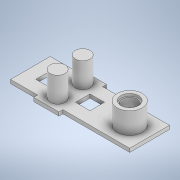
# Autodesk Inventor part: VexLegoWidget2
Saved by Autodesk Inventor 2020 (Build 240168000, 168)
## iProperties
Created: 2020-02-28
Part Number: VexLegoWidget2
Material: Generic
Document SubType Name: Modeling
Designer: Luke
Density: 1 g/cm^3
Appearance: Default
Author: Luke
Autodesk Inventor part; units mm, degrees
ref_plane "YZ Plane" through (0, 0, 0) normal (1, 0, 0) x (0, 1, 0)
ref_plane "XZ Plane" through (0, 0, 0) normal (0, 1, 0) x (-1, 0, 0)
ref_plane "XY Plane" through (0, 0, 0) normal (0, 0, 1) x (1, 0, 0)
sketch "Sketch4" plane through (0, 0, 0) normal (0, 1, 0) x (-1, 0, 0)
  line L0 (-19.05, 6.35) -> (2.3114, 6.35)
  line L1 (19.05, 6.35) -> (19.05, -6.35)
  line L2 (19.05, -6.35) -> (10.3886, -6.35)
  line L3 (-19.05, -6.35) -> (-19.05, 6.35)
  line L4 (-19.05, 6.35) -> (19.05, -6.35) construction
  line L5 (19.05, 6.35) -> (-19.05, -6.35) construction
  line L6 (-2.3114, 2.3114) -> (2.3114, 2.3114)
  line L7 (2.3114, 2.3114) -> (2.3114, -2.3114)
  line L8 (2.3114, -2.3114) -> (-2.3114, -2.3114)
  line L9 (-2.3114, -2.3114) -> (-2.3114, 2.3114)
  line L10 (-2.3114, 2.3114) -> (2.3114, -2.3114) construction
  line L11 (2.3114, 2.3114) -> (-2.3114, -2.3114) construction
  line L12 (10.3886, 2.3114) -> (15.0114, 2.3114)
  line L13 (15.0114, 2.3114) -> (15.0114, -2.3114)
  line L14 (15.0114, -2.3114) -> (10.3886, -2.3114)
  line L15 (10.3886, -2.3114) -> (10.3886, 2.3114)
  line L16 (10.3886, 2.3114) -> (15.0114, -2.3114) construction
  line L17 (15.0114, 2.3114) -> (10.3886, -2.3114) construction
  line L18 (10.3886, 6.35) -> (10.3886, 7.62)
  line L19 (2.3114, 6.35) -> (2.3114, 7.62)
  line L20 (2.3114, 7.62) -> (10.3886, 7.62)
  line L21 (10.3886, -6.35) -> (10.3886, -7.62)
  line L22 (2.3114, -6.35) -> (2.3114, -7.62)
  line L23 (2.3114, -7.62) -> (10.3886, -7.62)
  line L24 (10.3886, 6.35) -> (19.05, 6.35)
  line L25 (2.3114, -6.35) -> (-19.05, -6.35)
  point P0 (0, 0)
  point P1 (12.7, 0)
  dimension "d14" = 38.1
  dimension "d15" = 12.7
  dimension "d16" = 4.6228
  dimension "d17" = 4.6228
  dimension "d18" = 4.6228
  dimension "d19" = 12.7
  dimension "d20" = 1.27
  dimension "d27" = 1.27
  constraints: 52 end point, 9 parallel, 6 midpoint, 6 perpendicular, 4 horizontal, 4 vertical, 1 point on line
  measures "d14" distance of L1.end L3.start
  measures "d15" distance of L1.start L1.end
  measures "d16" distance of L7.end L8.end
  measures "d17" distance of L6.end L7.end
  measures "d18" distance of L13.end L14.end
  measures "d19" distance of point (0, 0) point (12.7, 0)
  measures "d20" distance of L18.start L18.end
  measures "d27" distance of L2.end L21.end
extrude "Extrusion2" add sketch "Sketch4" along normal blind 1.1684
sketch "Sketch5" plane through (0, 1.1684, 0) normal (0, 1, 0) x (1, 0, 0)
  circle A0 centre (-6.35, -4.0005) radius 2.3876
  point P0 (0, 0)
  point P1 (-6.35, 0)
  dimension "d24" = 6.35
  dimension "d25" = 4.7752
  dimension "d26" = 4.0005
  constraints: 1 centre point
  measures "d24" distance of point (0, 0) point (-6.35, 0)
  measures "d25" diameter of A0
  measures "d26" distance of point (-6.35, 0) A0.centre
sketch "Sketch6" plane through (0, 1.1684, 0) normal (0, 1, 0) x (1, 0, 0)
  circle A0 centre (-6.35, 4.0132) radius 2.3876
  point P0 (0, 0)
  point P1 (-6.35, 0)
  dimension "d29" = 6.35
  dimension "d30" = 4.7752
  dimension "d31" = 4.0132
  constraints: 1 centre point
  measures "d29" distance of point (0, 0) point (-6.35, 0)
  measures "d30" diameter of A0
  measures "d31" distance of A0.centre point (-6.35, 0)
extrude "Extrusion3" add sketch "Sketch5" along normal blind 8.001
extrude "Extrusion4" add sketch "Sketch6" along normal blind 8.001
sketch "Sketch8" plane through (0, 1.1684, 0) normal (0, 1, 0) x (1, 0, 0)
  circle A0 centre (12.7, 0) radius 4.0005
  point P0 (0, 0)
  dimension "d41" = 12.7
  dimension "d45" = 8.001
  constraints: 1 centre point, 1 coincident
  measures "d41" distance of point (12.7, 0) point (0, 0)
  measures "d45" diameter of A0
extrude "Extrusion6" add sketch "Sketch8" along normal blind 6.8326
sketch "Sketch9" plane through (12.7, 8.001, 0) normal (0, 1, 0) x (1, 0, 0)
  circle A0 centre (0, 0) radius 2.8067
  point P0 (-12.7, 0)
  dimension "d48" = 5.6134
  constraints: 1 centre point
  measures "d48" diameter of A0
extrude "Extrusion7" cut sketch "Sketch9" against normal blind 0.7874
sketch "Sketch10" plane through (12.7, 7.2136, 0) normal (0, 1, 0) x (1, 0, 0)
  circle A0 centre (0, 0) radius 2.4003
  point P0 (-12.7, 0)
  dimension "d51" = 4.8006
  constraints: 1 centre point
  measures "d51" diameter of A0
extrude "Extrusion8" cut sketch "Sketch10" against normal through all
sketch "Sketch11" plane through (0, 0, 0) normal (0, -1, 0) x (1, 0, 0)
  circle A0 centre (12.7, 0) radius 4.0005 projected
  circle A1 centre (12.7, 0) radius 2.8067
  point P0 (0, 0)
  dimension "d54" = 12.7
  dimension "d55" = 5.6134
  constraints: 1 centre point, 1 coincident
  measures "d54" distance of point (0, 0) point (12.7, 0)
  measures "d55" diameter of A1
extrude "Extrusion9" cut sketch "Sketch11" against normal blind 0.7874 contours A1
body "Solid2"
